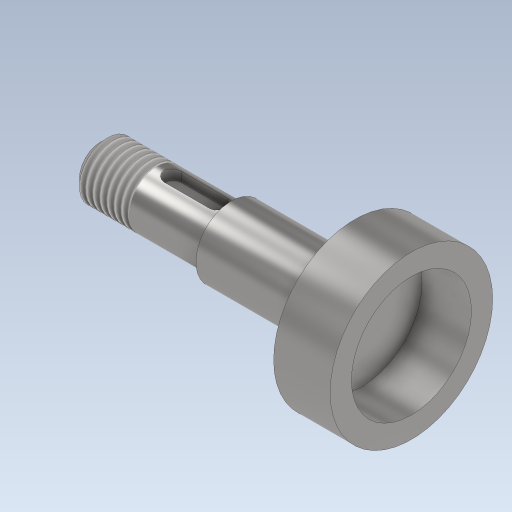
# Autodesk Inventor part: Pump-Motor-CW-Rotation:Cam Shaft
Saved by Autodesk Inventor 2024.2 (Build 282272000, 272)
## iProperties
Created: 2025-06-16
Material: Steel, Alloy
Document SubType Name: Modeling
Designer: cw
Density: 7.73 g/cm^3
Appearance: Semi-Polished
Author: cw
Autodesk Inventor part; units mm, degrees
ref_plane "YZ Plane" through (0, 0, 0) normal (1, 0, 0) x (0, 1, 0)
ref_plane "XZ Plane" through (0, 0, 0) normal (0, 1, 0) x (-1, 0, 0)
sketch "Sketch1" plane through (0, 0, 0) normal (0, 0, 1) x (1, 0, 0)
  line L0 (0, 0) -> (88, 0)
  line L1 (88, 0) -> (88, 23)
  line L2 (88, 23) -> (72, 23)
  line L3 (72, 23) -> (72, 10)
  line L4 (72, 10) -> (37, 10)
  line L5 (37, 10) -> (37, 8)
  line L6 (37, 8) -> (0, 8)
  line L7 (0, 8) -> (0, 0)
  line L8 (88, 17) -> (74, 17)
  line L9 (74, 17) -> (74, 0)
  dimension "d0" = 88
  dimension "d1" = 16
  dimension "d2" = 35
  dimension "d3" = 2
  dimension "d4" = 46
  dimension "d5" = 6
  dimension "d6" = 20
  dimension "d7" = 16
  constraints: 20 end point, 8 perpendicular, 2 horizontal, 2 point on line
  measures "d0" distance of L0.start L0.end
  measures "d1" distance of L1.end L2.end
  measures "d2" distance of L3.end L4.end
  measures "d3" distance between parallel lines of L9 L3
  measures "d4" diameter of L2 L0
  measures "d5" distance between parallel lines of L2 L8
  measures "d6" diameter of L4 L0
  measures "d7" diameter of L6 L0
revolve "Revolution1" add sketch "Sketch1" angle 360 about axis through (0, 0, 0) along (1, 0, 0) contours L7 L6 L5 L4 L3 L2 L1 L8 L9 L0
thread "Thread1" size "M16x2" class "6g" standard "ISO Metric profile" length 16
ref_plane "Work Plane1" through (18.5, 0, 8) normal (0, 0, 1) x (1, 0, 0)
sketch "Sketch2" plane through (18.5, 0, 8) normal (0, 0, 1) x (1, 0, 0)
  line L0 (-36.1, 0) -> (87.1, 0) construction
  line L1 (17.5, 0) -> (-0.5, 0) construction
  line L2 (15, -2.5) -> (2, -2.5)
  line L3 (2, 2.5) -> (15, 2.5)
  arc A0 (15, -2.5) -> (15, 2.5) centre (15, 0) ccw
  arc A1 (2, 2.5) -> (2, -2.5) centre (2, 0) ccw
  line L4 (18.5, -10) -> (18.5, 10) projected
  point P0 (-18.5, 0)
  point P1 (8.5, 0)
  point P2 (17.5, 0)
  point P3 (-0.5, 0)
  dimension "d11" = 5
  dimension "d12" = 18
  dimension "d13" = 1
  constraints: 8 end point, 8 point on circle, 4 point on line, 4 tangent, 2 centre point, 1 midpoint, 1 parallel
  measures "d11" distance between parallel lines of L2 L3
  measures "d12" distance of point (17.5, 0) point (-0.5, 0)
  measures "d13" distance from line of L4 L1.start
extrude "Extrusion1" cut sketch "Sketch2" against normal blind 3
chamfer "Chamfer1" distance 2 angle 45 1 edges at (0, -8, 0)
body "Solid1"
